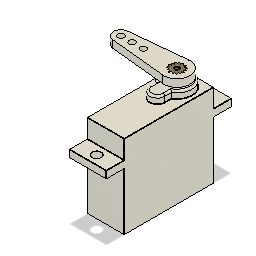
8g HS-45HB Servo v12 (Autodesk Fusion 360 design; units mm, degrees)
Autodesk Fusion 360 part; units mm, degrees
note: some values were not read from the file. Chosen so that the rebuilt part matches the saved one: which face or edge a step refers to. Set by a fixed rule: which sketch regions a step uses.
sketch "Sketch1" plane through (0, 0, 0) normal (0, 1, 0) x (1, 0, 0)
  line L0 (0, 0) -> (9.96, 0)
  line L1 (9.96, 0) -> (9.96, 23.99)
  line L2 (9.96, 23.99) -> (0, 23.99)
  line L3 (0, 23.99) -> (0, 0)
  dimension "d1" = 9.96
  dimension "d2" = 23.99
  dimension "d27" = 10
  measures "d1" distance of L0.start L0.end
  measures "d2" distance of L0.start L2.end
extrude "Extrude1" add sketch "Sketch1" along normal blind 22.35 makes body 1
sketch "Sketch2" plane through (0, 22.35, 0) normal (0, 1, 0) x (-1, 0, 0)
  line L0 (0, -23.99) -> (0, 0)
  line L1 (0, 0) -> (-9.96, 0)
  line L2 (-9.96, 0) -> (-9.96, -23.99)
  line L3 (-9.96, -23.99) -> (0, -23.99)
  line L4 (-4.98, -0.3366) -> (-4.98, -23.99) construction
  circle A0 centre (-4.98, -19.09) radius 4
  line L5 (-4.98, -23.09) -> (-4.98, -11.84)
  line L6 (-4.98, -11.84) -> (-4.98, -11.84)
  line L7 (-2.98, -13.84) -> (-2.98, -15.6259)
  line L8 (-4.98, -18.3366) -> (-4.98, -11.84)
  line L9 (-4.98, -11.84) -> (-4.98, -11.84)
  line L10 (-6.98, -13.84) -> (-6.98, -15.6259)
  line L11 (-4.98, -18.3366) -> (-4.98, -11.84)
  arc A1 (-2.98, -13.84) -> (-4.98, -11.84) centre (-4.98, -13.84) ccw
  arc A2 (-4.98, -11.84) -> (-6.98, -13.84) centre (-4.98, -13.84) ccw
  point P0 (-2.98, -11.84)
  point P1 (-6.98, -11.84)
  dimension "d5" = 8
  dimension "d6" = 11.25
  dimension "d7" = 6.4966
  dimension "d8" = 2
  dimension "d9" = 6.4966
  dimension "d10" = 2
  dimension "d11" = 2
  dimension "d12" = 2
  dimension "d31" = 4.9
  measures "d5" diameter of A0
  measures "d6" distance of L5.start L5.end
  measures "d7" distance of L5.end L8.start
  measures "d8" distance of L5.end P0
  measures "d9" distance of L5.end L8.start
  measures "d10" distance of L5.end P1
  measures "d11" radius of A1
  measures "d12" radius of A2
  measures "d31" distance of L3 A0.centre
extrude "Extrude2" add sketch "Sketch2" along normal blind 1.93 contours A0 L5 L8 L11 | A0 L5 L7 L8 L11 A1 | A0 L5 L8 L11 | A0 L5 L8 L10 L11 A2 bodies 1
fillet "Fillet1" radius 0.5 4 edges at (2.98, 24.28, -14.7329) (4.98, 24.28, -11.84) (6.98, 24.28, -14.7329) (4.98, 24.28, -23.09) on bodies 1
sketch "Sketch3" plane through (0, 0, -23.99) normal (0, 0, -1) x (-1, 0, 0)
  line L0 (-9.96, 0) -> (0, 0)
  line L1 (0, 0) -> (0, 22.35)
  line L2 (0, 22.35) -> (-9.96, 22.35)
  line L3 (-9.96, 22.35) -> (-9.96, 0)
  line L4 (-9.96, 17.35) -> (0, 17.35)
  line L5 (0, 17.35) -> (0, 15.35)
  line L6 (0, 15.35) -> (-9.96, 15.35)
  line L7 (-9.96, 15.35) -> (-9.96, 17.35)
  dimension "d16" = 2
  dimension "d28" = 7
  measures "d16" distance of L4 L6
  measures "d28" distance of L1.end L6
extrude "Extrude3" add sketch "Sketch3" along normal blind 4.805 contours L1 L3 L4 L5 L6 L7 bodies 1
sketch "Sketch4" plane through (0, 0, 0) normal (0, 0, 1) x (1, 0, 0)
  line L0 (0, 0) -> (9.96, 0)
  line L1 (9.96, 0) -> (9.96, 22.35)
  line L2 (9.96, 22.35) -> (0, 22.35)
  line L3 (0, 22.35) -> (0, 0)
  line L4 (9.96, 15.35) -> (0, 15.35)
  line L5 (0, 15.35) -> (0, 17.35)
  line L6 (0, 17.35) -> (9.96, 17.35)
  line L7 (9.96, 17.35) -> (9.96, 15.35)
extrude "Extrude4" add sketch "Sketch4" along normal blind 4.805 contours L1 L3 L4 L5 L6 L7 bodies 1
sketch "Sketch5" plane through (0, 17.35, 0) normal (0, 1, 0) x (-1, 0, 0)
  line L0 (0, -23.99) -> (-9.96, -23.99)
  line L1 (-9.96, -23.99) -> (-9.96, -28.795)
  line L2 (-9.96, -28.795) -> (0, -28.795)
  line L3 (0, -28.795) -> (0, -23.99)
  line L4 (-4.98, -28.795) -> (-4.98, -23.99)
  line L5 (0, 0) -> (-9.96, 0)
  line L6 (-9.96, 4.805) -> (0, 4.805)
  line L7 (-4.98, 0) -> (-4.98, 4.805)
  point P0 (-4.98, 2.4025)
  point P1 (-4.98, -26.3925)
hole "Hole1" at (4.98, 17.35, -26.3925) at (4.98, 17.35, 2.4025) direction (0, -1, 0) diameter 2.4 depth 11 tip angle 118 bodies 1
sketch "Sketch6" plane through (0, 24.28, 0) normal (0, 1, 0) x (-1, 0, 0)
  arc A0 (-6.48, -15.9277) -> (-3.48, -15.9277) centre (-4.98, -19.09) ccw
  line L0 (-3.48, -15.9277) -> (-3.48, -13.84)
  arc A1 (-3.48, -13.84) -> (-6.48, -13.84) centre (-4.98, -13.84) ccw
  line L1 (-6.48, -13.84) -> (-6.48, -15.9277)
  circle A2 centre (-4.98, -19.09) radius 2
  circle A3 centre (-4.98, -19.09) radius 1.5
  dimension "d25" = 4
  dimension "d26" = 3
  measures "d25" diameter of A2
  measures "d26" diameter of A3
extrude "Extrude1'" add sketch "Sketch6" along normal blind 2.43 separate body contours A2 | A3 makes body 2 in component "Gear"
sketch "Sketch7" plane through (0, 26.71, 0) normal (0, 1, 0) x (-1, 0, 0)
  circle A0 centre (-4.98, -19.09) radius 2
  circle A1 centre (-4.98, -19.09) radius 0.5
  circle A2 centre (-4.98, -19.09) radius 1.5
  line L0 (-4.98, -19.09) -> (-3.48, -19.09) construction
  line L1 (-4.98, -19.09) -> (-3.6097, -19.7001) construction
  line L2 (-4.98, -19.09) -> (-3.48, -19.09) construction
  arc A3 (-3.1529, -19.9035) -> (-2.98, -19.09) centre (-4.98, -19.09) ccw construction
  line L3 (-3.0237, -19.5058) -> (-3.48, -19.09)
  line L4 (-3.0237, -19.5058) -> (-3.6097, -19.7001)
  line L5 (-3.0237, -18.6742) -> (-3.48, -19.09)
  line L6 (-3.0237, -18.6742) -> (-3.6097, -18.4799)
  line L7 (-3.362, -17.9144) -> (-3.6097, -18.4799)
  line L8 (-3.362, -17.9144) -> (-3.9763, -17.9753)
  line L9 (-3.98, -17.3579) -> (-3.9763, -17.9753)
  line L10 (-3.98, -17.3579) -> (-4.5165, -17.6634)
  line L11 (-4.7709, -17.101) -> (-4.5165, -17.6634)
  line L12 (-4.7709, -17.101) -> (-5.1368, -17.5982)
  line L13 (-5.598, -17.1879) -> (-5.1368, -17.5982)
  line L14 (-5.598, -17.1879) -> (-5.73, -17.791)
  line L15 (-6.3183, -17.6037) -> (-5.73, -17.791)
  line L16 (-6.3183, -17.6037) -> (-6.1935, -18.2083)
  line L17 (-6.8071, -18.2765) -> (-6.1935, -18.2083)
  line L18 (-6.8071, -18.2765) -> (-6.4472, -18.7781)
  line L19 (-6.98, -19.09) -> (-6.4472, -18.7781)
  line L20 (-6.98, -19.09) -> (-6.4472, -19.4019)
  line L21 (-6.8071, -19.9035) -> (-6.4472, -19.4019)
  line L22 (-6.8071, -19.9035) -> (-6.1935, -19.9717)
  line L23 (-6.3183, -20.5763) -> (-6.1935, -19.9717)
  line L24 (-6.3183, -20.5763) -> (-5.73, -20.389)
  line L25 (-5.598, -20.9921) -> (-5.73, -20.389)
  line L26 (-5.598, -20.9921) -> (-5.1368, -20.5818)
  line L27 (-4.7709, -21.079) -> (-5.1368, -20.5818)
  line L28 (-4.7709, -21.079) -> (-4.5165, -20.5166)
  line L29 (-3.98, -20.8221) -> (-4.5165, -20.5166)
  line L30 (-3.98, -20.8221) -> (-3.9763, -20.2047)
  line L31 (-3.362, -20.2656) -> (-3.9763, -20.2047)
  line L32 (-3.362, -20.2656) -> (-3.6097, -19.7001)
  dimension "d32" = 1
  dimension "d33" = 3
  dimension "d34" = 2
  dimension "d35" = 24
  dimension "d37" = 360
  measures "d32" diameter of A1
  measures "d33" diameter of A2
  measures "d34" distance of A0.centre A3.start
  measures "d35" angle of L1 L2
chamfer "Chamfer1" distance 0.05 angle 45 2 edges at (6.8447, 26.71, -19.8132) (6.8447, 24.28, -19.8132) on bodies 2 in component "Gear"
extrude "Extrude2'" cut sketch "Sketch7" against normal blind 2.43 contours A0 L3 L5 | A0 L6 L7 | A0 L4 L32 | A0 L8 L9 | A0 L30 L31 | A0 L10 L11 | A0 L28 L29 | A0 L12 L13 | A0 L26 L27 | A0 L14 L15 | A0 L24 L25 | A0 L16 L17 | A0 L22 L23 | A0 L18 L19 | A0 L20 L21 bodies 2 in component "Gear"
sketch "Sketch8" plane through (0, 26.71, 0) normal (0, 1, 0) x (-1, 0, 0)
  line L0 (-4.0306, -17.3867) -> (-4.5165, -17.6634)
  line L1 (-4.5165, -17.6634) -> (-4.747, -17.154)
  arc A0 (-4.747, -17.154) -> (-4.8054, -17.1478) centre (-4.98, -19.09) ccw
  line L2 (-4.8054, -17.1478) -> (-5.1368, -17.5982)
  line L3 (-5.1368, -17.5982) -> (-5.5546, -17.2266)
  arc A1 (-5.5546, -17.2266) -> (-5.6105, -17.2447) centre (-4.98, -19.09) ccw
  line L4 (-5.6105, -17.2447) -> (-5.73, -17.791)
  line L5 (-5.73, -17.791) -> (-6.2628, -17.6214)
  arc A2 (-6.2628, -17.6214) -> (-6.3065, -17.6607) centre (-4.98, -19.09) ccw
  line L6 (-6.3065, -17.6607) -> (-6.1935, -18.2083)
  line L7 (-6.1935, -18.2083) -> (-6.7493, -18.2701)
  arc A3 (-6.7493, -18.2701) -> (-6.7732, -18.3238) centre (-4.98, -19.09) ccw
  line L8 (-6.7732, -18.3238) -> (-6.4472, -18.7781)
  line L9 (-6.4472, -18.7781) -> (-6.9298, -19.0606)
  arc A4 (-6.9298, -19.0606) -> (-6.9298, -19.1194) centre (-4.98, -19.09) ccw
  line L10 (-6.9298, -19.1194) -> (-6.4472, -19.4019)
  line L11 (-6.4472, -19.4019) -> (-6.7732, -19.8562)
  arc A5 (-6.7732, -19.8562) -> (-6.7493, -19.9099) centre (-4.98, -19.09) ccw
  line L12 (-6.7493, -19.9099) -> (-6.1935, -19.9717)
  line L13 (-6.1935, -19.9717) -> (-6.3065, -20.5193)
  arc A6 (-6.3065, -20.5193) -> (-6.2628, -20.5586) centre (-4.98, -19.09) ccw
  line L14 (-6.2628, -20.5586) -> (-5.73, -20.389)
  line L15 (-5.73, -20.389) -> (-5.6105, -20.9353)
  arc A7 (-5.6105, -20.9353) -> (-5.5546, -20.9534) centre (-4.98, -19.09) ccw
  line L16 (-5.5546, -20.9534) -> (-5.1368, -20.5818)
  line L17 (-5.1368, -20.5818) -> (-4.8054, -21.0322)
  arc A8 (-4.8054, -21.0322) -> (-4.747, -21.026) centre (-4.98, -19.09) ccw
  line L18 (-4.747, -21.026) -> (-4.5165, -20.5166)
  line L19 (-4.5165, -20.5166) -> (-4.0306, -20.7933)
  arc A9 (-4.0306, -20.7933) -> (-3.9797, -20.7639) centre (-4.98, -19.09) ccw
  line L20 (-3.9797, -20.7639) -> (-3.9763, -20.2047)
  line L21 (-3.9763, -20.2047) -> (-3.4199, -20.2598)
  arc A10 (-3.4199, -20.2598) -> (-3.3853, -20.2123) centre (-4.98, -19.09) ccw
  line L22 (-3.3853, -20.2123) -> (-3.6097, -19.7001)
  line L23 (-3.6097, -19.7001) -> (-3.0789, -19.5241)
  arc A11 (-3.0789, -19.5241) -> (-3.0667, -19.4666) centre (-4.98, -19.09) ccw
  line L24 (-3.0667, -19.4666) -> (-3.48, -19.09)
  line L25 (-3.48, -19.09) -> (-3.0667, -18.7134)
  arc A12 (-3.0667, -18.7134) -> (-3.0789, -18.6559) centre (-4.98, -19.09) ccw
  line L26 (-3.0789, -18.6559) -> (-3.6097, -18.4799)
  line L27 (-3.6097, -18.4799) -> (-3.3853, -17.9677)
  arc A13 (-3.3853, -17.9677) -> (-3.4199, -17.9202) centre (-4.98, -19.09) ccw
  line L28 (-3.4199, -17.9202) -> (-3.9763, -17.9753)
  line L29 (-3.9763, -17.9753) -> (-3.9797, -17.4161)
  arc A14 (-3.9797, -17.4161) -> (-4.0306, -17.3867) centre (-4.98, -19.09) ccw
  point P0 (-4.98, -19.09)
hole "Hole1'" at (4.98, 26.71, -19.09) direction (0, -1, 0) diameter 0.769 depth 1 tip angle 118 counterbore diameter 1.2 counterbore depth 0.1 bodies 2 in component "Gear"
thread "Thread1" "ISO Metric profile 1.0 M1x0.25 6H" in component "Gear"
copy_body "Body->Comp1" bodies 1 removing the originals makes body 3 in component "Body"
fillet "Fillet1'" radius 0.1 40 edges at (4.98, 22.35, -11.84) (2.98, 22.35, -14.7329) (0, 22.35, -11.995) (4.98, 22.35, 0) (9.96, 22.35, -11.995) (4.98, 22.35, -23.99) (4.98, 22.35, -23.09) (6.98, 22.35, -14.7329) (0, 7.675, -23.99) (0, 15.35, -26.3925) (0, 16.35, -28.795) (0, 17.35, -26.3925) (0, 19.85, -23.99) (0, 19.85, 0) (0, 17.35, 2.4025) (0, 16.35, 4.805) (0, 15.35, 2.4025) (0, 7.675, 0) (0, 0, -11.995) (4.98, 17.35, 0) (9.96, 19.85, 0) (9.96, 7.675, 0) (9.96, 15.35, 2.4025) (9.96, 16.35, 4.805) (9.96, 17.35, 2.4025) (9.96, 19.85, -23.99) (9.96, 17.35, -26.3925) (9.96, 16.35, -28.795) (9.96, 15.35, -26.3925) (9.96, 7.675, -23.99) (9.96, 0, -11.995) (4.98, 17.35, -23.99) (4.98, 0, -23.99) (4.98, 15.35, -23.99) (4.98, 15.35, -28.795) (4.98, 17.35, -28.795) (4.98, 17.35, 4.805) (4.98, 15.35, 4.805) (4.98, 15.35, 0) (4.98, 0, 0) on bodies 3 in component "Body"
sketch "Sketch9" plane through (0, 0, -23.99) normal (0, 0, -1) x (-1, 0, 0)
  line L0 (-9.86, 0.1) -> (-0.1, 0.1)
  line L1 (-0.1, 0.1) -> (-0.1, 15.25)
  line L2 (-0.1, 15.25) -> (-9.86, 15.25)
  line L3 (-9.86, 15.25) -> (-9.86, 0.1)
  line L4 (-9.86, 0) -> (-0.1, 0)
  line L5 (-4.98, 0) -> (-4.98, 2)
  circle A0 centre (-4.98, 2) radius 0.5
  line L6 (-4.98, 2) -> (-3.98, 2)
  line L7 (-4.98, 2) -> (-5.98, 2)
  circle A1 centre (-3.98, 2) radius 0.5
  circle A2 centre (-5.98, 2) radius 0.5
  dimension "d45" = 2
  dimension "d46" = 1
  dimension "d47" = 1
  dimension "d48" = 1
  measures "d45" distance of L5.start L5.end
  measures "d46" diameter of A0
  measures "d47" distance of L5.end L6.end
  measures "d48" distance of L5.end L7.end
extrude "Extrude5" add sketch "Sketch9" along normal blind 3 separate body contours L5 A0 L7 | A2 | A1 | L5 A0 L6 | A0 L6 L7 makes body 4 at (4.3108, 2.3749, -24.99)
copy_body "Body->Comp2" bodies 4 removing the originals makes body 5 in component "Wires"
fillet "Fillet1''" radius 0.05 15 edges at (3.362, 25.495, -20.2656) (3.0237, 25.495, -19.5058) (3.0237, 25.495, -18.6742) (3.362, 25.495, -17.9144) (3.98, 25.495, -17.3579) (4.7709, 25.495, -17.101) (5.598, 25.495, -17.1879) (3.98, 25.495, -20.8221) (4.7709, 25.495, -21.079) (5.598, 25.495, -20.9921) (6.3183, 25.495, -20.5763) (6.8071, 25.495, -19.9035) (6.98, 25.495, -19.09) (6.8071, 25.495, -18.2765) (6.3183, 25.495, -17.6037) on bodies 2 in component "Gear"
chamfer "Chamfer2" distance 0.04 angle 45 2 edges at (5.197, 26.61, -19.6494) (5.1191, 26.61, -19.4487) on bodies 2 in component "Gear"
fillet "Fillet2" radius 0.03 1 edges at (5.197, 26.71, -19.6494) on bodies 2 in component "Gear"
fillet "Fillet2'" radius 0.05 4 edges at (5.4139, 17.35, -27.5113) (4.5461, 15.35, -27.5113) (5.4139, 17.35, 1.2837) (4.5461, 15.35, 1.2837) on bodies 3 in component "Body"
sketch "Sketch10" plane through (0, 26.71, 0) normal (0, 1, 0) x (-1, 0, 0)
  arc A0 (-6.2924, -17.6477) -> (-6.301, -17.6874) centre (-6.252, -17.6773) ccw
  line L0 (-6.301, -17.6874) -> (-6.1935, -18.2083)
  line L1 (-6.1935, -18.2083) -> (-6.7222, -18.2671)
  arc A1 (-6.7222, -18.2671) -> (-6.7572, -18.2876) centre (-6.7167, -18.3168) ccw
  arc A2 (-6.7572, -18.2876) -> (-6.7655, -18.3062) centre (-4.98, -19.09) ccw
  arc A3 (-6.7655, -18.3062) -> (-6.7573, -18.3459) centre (-6.7167, -18.3168) ccw
  line L2 (-6.7573, -18.3459) -> (-6.4472, -18.7781)
  line L3 (-6.4472, -18.7781) -> (-6.9063, -19.0468)
  arc A4 (-6.9063, -19.0468) -> (-6.93, -19.0798) centre (-6.881, -19.09) ccw
  arc A5 (-6.93, -19.0798) -> (-6.93, -19.1002) centre (-4.98, -19.09) ccw
  arc A6 (-6.93, -19.1002) -> (-6.9063, -19.1332) centre (-6.881, -19.09) ccw
  line L4 (-6.9063, -19.1332) -> (-6.4472, -19.4019)
  line L5 (-6.4472, -19.4019) -> (-6.7573, -19.8341)
  arc A7 (-6.7573, -19.8341) -> (-6.7655, -19.8738) centre (-6.7167, -19.8632) ccw
  arc A8 (-6.7655, -19.8738) -> (-6.7572, -19.8924) centre (-4.98, -19.09) ccw
  arc A9 (-6.7572, -19.8924) -> (-6.7222, -19.9129) centre (-6.7167, -19.8632) ccw
  line L6 (-6.7222, -19.9129) -> (-6.1935, -19.9717)
  line L7 (-6.1935, -19.9717) -> (-6.301, -20.4926)
  arc A10 (-6.301, -20.4926) -> (-6.2924, -20.5323) centre (-6.252, -20.5027) ccw
  arc A11 (-6.2924, -20.5323) -> (-6.2772, -20.5459) centre (-4.98, -19.09) ccw
  arc A12 (-6.2772, -20.5459) -> (-6.2369, -20.5504) centre (-6.252, -20.5027) ccw
  line L8 (-6.2369, -20.5504) -> (-5.73, -20.389)
  line L9 (-5.73, -20.389) -> (-5.6163, -20.9087)
  arc A13 (-5.6163, -20.9087) -> (-5.5923, -20.9414) centre (-5.5674, -20.898) ccw
  arc A14 (-5.5923, -20.9414) -> (-5.5729, -20.9477) centre (-4.98, -19.09) ccw
  arc A15 (-5.5729, -20.9477) -> (-5.5342, -20.9353) centre (-5.5674, -20.898) ccw
  line L10 (-5.5342, -20.9353) -> (-5.1368, -20.5818)
  line L11 (-5.1368, -20.5818) -> (-4.8216, -21.0102)
  arc A16 (-4.8216, -21.0102) -> (-4.7863, -21.0304) centre (-4.7813, -20.9806) ccw
  arc A17 (-4.7863, -21.0304) -> (-4.766, -21.0282) centre (-4.98, -19.09) ccw
  arc A18 (-4.766, -21.0282) -> (-4.7357, -21.0012) centre (-4.7813, -20.9806) ccw
  line L12 (-4.7357, -21.0012) -> (-4.5165, -20.5166)
  line L13 (-4.5165, -20.5166) -> (-4.0542, -20.7798)
  arc A19 (-4.0542, -20.7798) -> (-4.0138, -20.7838) centre (-4.0295, -20.7363) ccw
  arc A20 (-4.0138, -20.7838) -> (-3.9962, -20.7736) centre (-4.98, -19.09) ccw
  arc A21 (-3.9962, -20.7736) -> (-3.9795, -20.7366) centre (-4.0295, -20.7363) ccw
  line L14 (-3.9795, -20.7366) -> (-3.9763, -20.2047)
  line L15 (-3.9763, -20.2047) -> (-3.447, -20.2572)
  arc A22 (-3.447, -20.2572) -> (-3.4084, -20.2444) centre (-3.442, -20.2074) ccw
  arc A23 (-3.4084, -20.2444) -> (-3.3964, -20.2279) centre (-4.98, -19.09) ccw
  arc A24 (-3.3964, -20.2279) -> (-3.3962, -20.1873) centre (-3.442, -20.2074) ccw
  line L16 (-3.3962, -20.1873) -> (-3.6097, -19.7001)
  line L17 (-3.6097, -19.7001) -> (-3.1048, -19.5327)
  arc A25 (-3.1048, -19.5327) -> (-3.0748, -19.5054) centre (-3.1205, -19.4852) ccw
  arc A26 (-3.0748, -19.5054) -> (-3.0705, -19.4854) centre (-4.98, -19.09) ccw
  arc A27 (-3.0705, -19.4854) -> (-3.0868, -19.4483) centre (-3.1205, -19.4852) ccw
  line L18 (-3.0868, -19.4483) -> (-3.48, -19.09)
  line L19 (-3.48, -19.09) -> (-3.0868, -18.7317)
  arc A28 (-3.0868, -18.7317) -> (-3.0705, -18.6946) centre (-3.1205, -18.6948) ccw
  arc A29 (-3.0705, -18.6946) -> (-3.0748, -18.6746) centre (-4.98, -19.09) ccw
  arc A30 (-3.0748, -18.6746) -> (-3.1048, -18.6473) centre (-3.1205, -18.6948) ccw
  line L20 (-3.1048, -18.6473) -> (-3.6097, -18.4799)
  line L21 (-3.6097, -18.4799) -> (-3.3962, -17.9927)
  arc A31 (-3.3962, -17.9927) -> (-3.3964, -17.9521) centre (-3.442, -17.9726) ccw
  arc A32 (-3.3964, -17.9521) -> (-3.4084, -17.9356) centre (-4.98, -19.09) ccw
  arc A33 (-3.4084, -17.9356) -> (-3.447, -17.9228) centre (-3.442, -17.9726) ccw
  line L22 (-3.447, -17.9228) -> (-3.9763, -17.9753)
  line L23 (-3.9763, -17.9753) -> (-3.9795, -17.4434)
  arc A34 (-3.9795, -17.4434) -> (-3.9962, -17.4064) centre (-4.0295, -17.4437) ccw
  arc A35 (-3.9962, -17.4064) -> (-4.0138, -17.3962) centre (-4.98, -19.09) ccw
  arc A36 (-4.0138, -17.3962) -> (-4.0542, -17.4002) centre (-4.0295, -17.4437) ccw
  line L24 (-4.0542, -17.4002) -> (-4.5165, -17.6634)
  line L25 (-4.5165, -17.6634) -> (-4.7357, -17.1788)
  arc A37 (-4.7357, -17.1788) -> (-4.766, -17.1518) centre (-4.7813, -17.1994) ccw
  arc A38 (-4.766, -17.1518) -> (-4.7863, -17.1496) centre (-4.98, -19.09) ccw
  arc A39 (-4.7863, -17.1496) -> (-4.8216, -17.1698) centre (-4.7813, -17.1994) ccw
  line L26 (-4.8216, -17.1698) -> (-5.1368, -17.5982)
  line L27 (-5.1368, -17.5982) -> (-5.5342, -17.2447)
  arc A40 (-5.5342, -17.2447) -> (-5.5729, -17.2323) centre (-5.5674, -17.282) ccw
  arc A41 (-5.5729, -17.2323) -> (-5.5923, -17.2386) centre (-4.98, -19.09) ccw
  arc A42 (-5.5923, -17.2386) -> (-5.6163, -17.2713) centre (-5.5674, -17.282) ccw
  line L28 (-5.6163, -17.2713) -> (-5.73, -17.791)
  line L29 (-5.73, -17.791) -> (-6.2369, -17.6296)
  arc A43 (-6.2369, -17.6296) -> (-6.2772, -17.6341) centre (-6.252, -17.6773) ccw
  arc A44 (-6.2772, -17.6341) -> (-6.2924, -17.6477) centre (-4.98, -19.09) ccw
  circle A45 centre (-4.98, -19.09) radius 0.63
sketch "Sketch11" plane through (0, 26.71, 0) normal (0, 1, 0) x (-1, 0, 0)
  circle A0 centre (-4.98, -19.09) radius 3.5
  line L0 (-4.98, -15.59) -> (-4.98, -22.59)
  line L1 (-4.98, -19.09) -> (10.02, -19.09)
  circle A1 centre (10.02, -19.09) radius 0.8255
  circle A2 centre (7.02, -19.09) radius 0.8255
  circle A3 centre (4.02, -19.09) radius 0.8255
  circle A4 centre (10.02, -19.09) radius 2
  line L2 (-4.63, -22.5725) -> (10.22, -21.08)
  line L3 (10.22, -17.1) -> (-4.63, -15.6075)
  arc A5 (-6.2369, -17.6296) -> (-6.2772, -17.6341) centre (-6.252, -17.6773) ccw
  spline S0 degree 3 poles (-6.2772, -17.6341) (-6.2802, -17.6358) (-6.283, -17.6378) (-6.288, -17.6424) (-6.2903, -17.645) (-6.2924, -17.6477) knots 0.008298 0.008298 0.008298 0.008298 0.009323 0.009323 0.010347 0.010347 0.010347 0.010347
  arc A6 (-6.2924, -17.6477) -> (-6.301, -17.6874) centre (-6.252, -17.6773) ccw
  line L4 (-6.2369, -17.6296) -> (-5.73, -17.791)
  arc A7 (-6.7222, -18.2671) -> (-6.7572, -18.2876) centre (-6.7167, -18.3168) ccw
  spline S1 degree 3 poles (-6.7572, -18.2876) (-6.7592, -18.2903) (-6.761, -18.2933) (-6.7637, -18.2996) (-6.7648, -18.3029) (-6.7655, -18.3062) knots 0.008298 0.008298 0.008298 0.008298 0.009323 0.009323 0.010347 0.010347 0.010347 0.010347
  arc A8 (-6.7655, -18.3062) -> (-6.7573, -18.3459) centre (-6.7167, -18.3168) ccw
  line L5 (-6.7222, -18.2671) -> (-6.1935, -18.2083)
  arc A9 (-6.9063, -19.0468) -> (-6.93, -19.0798) centre (-6.881, -19.09) ccw
  spline S2 degree 3 poles (-6.93, -19.0798) (-6.9307, -19.0831) (-6.931, -19.0866) (-6.931, -19.0934) (-6.9307, -19.0969) (-6.93, -19.1002) knots 0.008298 0.008298 0.008298 0.008298 0.009323 0.009323 0.010347 0.010347 0.010347 0.010347
  arc A10 (-6.93, -19.1002) -> (-6.9063, -19.1332) centre (-6.881, -19.09) ccw
  line L6 (-6.4472, -19.4019) -> (-6.9063, -19.1332)
  line L7 (-5.73, -17.791) -> (-5.6163, -17.2713)
  arc A11 (-5.5923, -17.2386) -> (-5.6163, -17.2713) centre (-5.5674, -17.282) ccw
  arc A12 (-5.5342, -17.2447) -> (-5.5729, -17.2323) centre (-5.5674, -17.282) ccw
  line L8 (-5.5342, -17.2447) -> (-5.1368, -17.5982)
  line L9 (-5.1368, -17.5982) -> (-4.8216, -17.1698)
  arc A13 (-4.7863, -17.1496) -> (-4.8216, -17.1698) centre (-4.7813, -17.1994) ccw
  arc A14 (-4.7357, -17.1788) -> (-4.766, -17.1518) centre (-4.7813, -17.1994) ccw
  line L10 (-4.7357, -17.1788) -> (-4.5165, -17.6634)
  line L11 (-4.5165, -17.6634) -> (-4.0542, -17.4002)
  arc A15 (-4.0138, -17.3962) -> (-4.0542, -17.4002) centre (-4.0295, -17.4437) ccw
  arc A16 (-3.9795, -17.4434) -> (-3.9962, -17.4064) centre (-4.0295, -17.4437) ccw
  line L12 (-3.9795, -17.4434) -> (-3.9763, -17.9753)
  line L13 (-3.9763, -17.9753) -> (-3.447, -17.9228)
  arc A17 (-3.4084, -17.9356) -> (-3.447, -17.9228) centre (-3.442, -17.9726) ccw
  arc A18 (-3.3962, -17.9927) -> (-3.3964, -17.9521) centre (-3.442, -17.9726) ccw
  line L14 (-3.3962, -17.9927) -> (-3.6097, -18.4799)
  line L15 (-3.6097, -18.4799) -> (-3.1048, -18.6473)
  arc A19 (-3.0748, -18.6746) -> (-3.1048, -18.6473) centre (-3.1205, -18.6948) ccw
  arc A20 (-3.0868, -18.7317) -> (-3.0705, -18.6946) centre (-3.1205, -18.6948) ccw
  line L16 (-3.0868, -18.7317) -> (-3.48, -19.09)
  line L17 (-3.48, -19.09) -> (-3.0868, -19.4483)
  arc A21 (-3.0705, -19.4854) -> (-3.0868, -19.4483) centre (-3.1205, -19.4852) ccw
  arc A22 (-3.1048, -19.5327) -> (-3.0748, -19.5054) centre (-3.1205, -19.4852) ccw
  line L18 (-3.1048, -19.5327) -> (-3.6097, -19.7001)
  line L19 (-3.6097, -19.7001) -> (-3.3962, -20.1873)
  arc A23 (-3.3964, -20.2279) -> (-3.3962, -20.1873) centre (-3.442, -20.2074) ccw
  arc A24 (-3.447, -20.2572) -> (-3.4084, -20.2444) centre (-3.442, -20.2074) ccw
  line L20 (-3.447, -20.2572) -> (-3.9763, -20.2047)
  line L21 (-3.9763, -20.2047) -> (-3.9795, -20.7366)
  arc A25 (-3.9962, -20.7736) -> (-3.9795, -20.7366) centre (-4.0295, -20.7363) ccw
  arc A26 (-4.0542, -20.7798) -> (-4.0138, -20.7838) centre (-4.0295, -20.7363) ccw
  line L22 (-4.0542, -20.7798) -> (-4.5165, -20.5166)
  line L23 (-4.5165, -20.5166) -> (-4.7357, -21.0012)
  arc A27 (-4.766, -21.0282) -> (-4.7357, -21.0012) centre (-4.7813, -20.9806) ccw
  arc A28 (-4.8216, -21.0102) -> (-4.7863, -21.0304) centre (-4.7813, -20.9806) ccw
  line L24 (-4.8216, -21.0102) -> (-5.1368, -20.5818)
  line L25 (-5.1368, -20.5818) -> (-5.5342, -20.9353)
  arc A29 (-5.5729, -20.9477) -> (-5.5342, -20.9353) centre (-5.5674, -20.898) ccw
  arc A30 (-5.6163, -20.9087) -> (-5.5923, -20.9414) centre (-5.5674, -20.898) ccw
  line L26 (-5.6163, -20.9087) -> (-5.73, -20.389)
  line L27 (-5.73, -20.389) -> (-6.2369, -20.5504)
  arc A31 (-6.2772, -20.5459) -> (-6.2369, -20.5504) centre (-6.252, -20.5027) ccw
  arc A32 (-6.301, -20.4926) -> (-6.2924, -20.5323) centre (-6.252, -20.5027) ccw
  line L28 (-6.301, -20.4926) -> (-6.1935, -19.9717)
  line L29 (-6.1935, -19.9717) -> (-6.7222, -19.9129)
  arc A33 (-6.7572, -19.8924) -> (-6.7222, -19.9129) centre (-6.7167, -19.8632) ccw
  arc A34 (-6.7573, -19.8341) -> (-6.7655, -19.8738) centre (-6.7167, -19.8632) ccw
  line L30 (-6.7573, -19.8341) -> (-6.4472, -19.4019)
  line L31 (-6.9063, -19.0468) -> (-6.4472, -18.7781)
  line L32 (-6.4472, -18.7781) -> (-6.7573, -18.3459)
  line L33 (-6.1935, -18.2083) -> (-6.301, -17.6874)
  spline S3 degree 3 poles (-6.7655, -19.8738) (-6.7648, -19.8771) (-6.7637, -19.8804) (-6.761, -19.8867) (-6.7592, -19.8897) (-6.7572, -19.8924) knots 0.008298 0.008298 0.008298 0.008298 0.009323 0.009323 0.010347 0.010347 0.010347 0.010347
  spline S4 degree 3 poles (-6.2924, -20.5323) (-6.2903, -20.535) (-6.288, -20.5376) (-6.283, -20.5422) (-6.2802, -20.5442) (-6.2772, -20.5459) knots 0.026329 0.026329 0.026329 0.026329 0.027353 0.027353 0.028378 0.028378 0.028378 0.028378
  spline S5 degree 3 poles (-5.5923, -20.9414) (-5.5893, -20.9431) (-5.5861, -20.9445) (-5.5797, -20.9466) (-5.5763, -20.9473) (-5.5729, -20.9477) knots 0.008298 0.008298 0.008298 0.008298 0.009323 0.009323 0.010347 0.010347 0.010347 0.010347
  spline S6 degree 3 poles (-4.7863, -21.0304) (-4.7829, -21.0307) (-4.7795, -21.0307) (-4.7727, -21.03) (-4.7693, -21.0293) (-4.766, -21.0282) knots 0.008298 0.008298 0.008298 0.008298 0.009323 0.009323 0.010347 0.010347 0.010347 0.010347
  spline S7 degree 3 poles (-4.0138, -20.7838) (-4.0106, -20.7828) (-4.0074, -20.7813) (-4.0015, -20.7779) (-3.9987, -20.7759) (-3.9962, -20.7736) knots 0.008298 0.008298 0.008298 0.008298 0.009323 0.009323 0.010347 0.010347 0.010347 0.010347
  spline S8 degree 3 poles (-5.5729, -17.2323) (-5.5763, -17.2327) (-5.5797, -17.2334) (-5.5861, -17.2355) (-5.5893, -17.2369) (-5.5923, -17.2386) knots 0.008298 0.008298 0.008298 0.008298 0.009323 0.009323 0.010347 0.010347 0.010347 0.010347
  spline S9 degree 3 poles (-4.766, -17.1518) (-4.7693, -17.1507) (-4.7727, -17.15) (-4.7795, -17.1493) (-4.7829, -17.1493) (-4.7863, -17.1496) knots 0.008298 0.008298 0.008298 0.008298 0.009323 0.009323 0.010347 0.010347 0.010347 0.010347
  spline S10 degree 3 poles (-3.9962, -17.4064) (-3.9987, -17.4041) (-4.0015, -17.4021) (-4.0074, -17.3987) (-4.0106, -17.3972) (-4.0138, -17.3962) knots 0.008298 0.008298 0.008298 0.008298 0.009323 0.009323 0.010347 0.010347 0.010347 0.010347
  spline S11 degree 3 poles (-3.3964, -17.9521) (-3.3978, -17.949) (-3.3996, -17.946) (-3.4036, -17.9405) (-3.4059, -17.9379) (-3.4084, -17.9356) knots 0.008298 0.008298 0.008298 0.008298 0.009323 0.009323 0.010347 0.010347 0.010347 0.010347
  spline S12 degree 3 poles (-3.0705, -18.6946) (-3.0705, -18.6911) (-3.0709, -18.6877) (-3.0723, -18.681) (-3.0734, -18.6777) (-3.0748, -18.6746) knots 0.008298 0.008298 0.008298 0.008298 0.009323 0.009323 0.010347 0.010347 0.010347 0.010347
  spline S13 degree 3 poles (-3.0748, -19.5054) (-3.0734, -19.5023) (-3.0723, -19.499) (-3.0709, -19.4923) (-3.0705, -19.4889) (-3.0705, -19.4854) knots 0.008298 0.008298 0.008298 0.008298 0.009323 0.009323 0.010347 0.010347 0.010347 0.010347
  spline S14 degree 3 poles (-3.4084, -20.2444) (-3.4059, -20.2421) (-3.4036, -20.2395) (-3.3996, -20.234) (-3.3978, -20.231) (-3.3964, -20.2279) knots 0.008298 0.008298 0.008298 0.008298 0.009323 0.009323 0.010347 0.010347 0.010347 0.010347
  point P0 (-4.98, -19.09)
  point P1 (7.02, -19.09)
  point P2 (4.02, -19.09)
  dimension "d69" = 7
  dimension "d70" = 15
  dimension "d71" = 1.651
  dimension "d74" = -3
  dimension "d75" = 0
  dimension "d76" = 4
  measures "d69" diameter of A0
  measures "d70" distance of P0 L1.end
  measures "d71" diameter of A1
  measures "d76" diameter of A4
extrude "Extrude1''" add sketch "Sketch11" against normal blind 2 separate body contours A0 L0 L1 L9 A13 A14 L10 L11 A15 A16 L12 L13 A17 A18 L14 L15 A19 A20 L16 S9 S10 S11 S12 | A0 L1 A2 A3 A4 L2 | A0 L0 L1 L17 A21 A22 L18 L19 A23 A24 L20 L21 A25 A26 L22 L23 A27 A28 L24 S6 S7 S13 S14 | A0 L1 A2 A3 A4 L3 | A0 L0 A5 S0 A6 L4 A7 S1 A8 L5 A9 S2 A10 L6 L7 A11 A12 L8 L9 L24 L25 A29 A30 L26 L27 A31 A32 L28 L29 A33 A34 L30 L31 L32 L33 S3 S4 S5 S8 | A4 makes body 6 in component "arm"
component "Gear" placed x (1, 0, 0) y (0, 1, 0) z (0, 0, 1) at (0, 0, 0)
component "Body" placed x (1, 0, 0) y (0, 1, 0) z (0, 0, 1) at (0, 0, 0)
component "Wires" placed x (1, 0, 0) y (0, 1, 0) z (0, 0, 1) at (0, 0, 0)
component "arm" placed x (1, 0, 0) y (0, 1, 0) z (0, 0, 1) at (0, 0, 0)
equation "d3 = 15.35 mm + 7 mm"
equation "d13 = 8.93 mm - 7 mm"
equation "d18 = ( ( 33.6 - 23.99 ) / 2 ) * 1 mm"
equation "d20 = ( ( 33.6 - 23.99 ) / 2 ) * 1 mm"
equation "d35 = ( 360 / 15 ) * 1 deg"
equation "d70 = last_hole_dist"
equation "d71 = 0.055 in + 0.01 in"
equation "last_hole_dist = 15 mm"
equation "holes = 7 mm"
